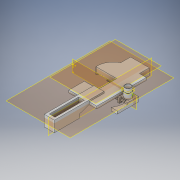
# Autodesk Inventor part: chuteandblocker20200305
Saved by Autodesk Inventor 2018 (Build 220112000, 112)
## iProperties
Created: 2017-08-23
Part Number: chuteandblocker20200305
Material: Generic
Document SubType Name: Modeling
Designer: Kim
Density: 1 g/cm^3
Appearance: Default
Author: Kim
Autodesk Inventor part; units mm, degrees
ref_plane "YZ Plane" through (0, 0, 0) normal (1, 0, 0) x (0, 1, 0)
ref_plane "XZ Plane" through (0, 0, 0) normal (0, 1, 0) x (-1, 0, 0)
ref_plane "XY Plane" through (0, 0, 0) normal (0, 0, 1) x (1, 0, 0)
sketch "Sketch1" plane through (0, 0, 0) normal (0, 1, 0) x (-1, 0, 0)
  line L0 (0, 24.7368) -> (-48.52, 24.7368)
  line L1 (-48.52, 24.7368) -> (-48.52, -25.1832)
  line L2 (-48.52, -25.1832) -> (0, -25.1832)
  line L3 (0, -25.1832) -> (0, 24.7368)
  point P0 (0, 0)
  dimension "d0" = 48.52
  dimension "d1" = 49.92
  constraints: 8 end point, 2 parallel, 1 horizontal, 1 perpendicular
  measures "d0" distance of L2.end L1.end
  measures "d1" distance of L1.end L0.end
extrude "Extrusion1" add sketch "Sketch1" along normal blind 2.5
sketch "Sketch2" plane through (0, 2.5, 0) normal (0, 1, 0) x (1, 0, 0)
  line L0 (0, 25.1832) -> (0, -24.7368) projected
  line L1 (0, -9.2266) -> (34.56, -9.2266)
  line L2 (34.56, -9.2266) -> (34.56, 9.3534)
  line L3 (34.56, 9.3534) -> (0, 9.3534)
  line L4 (0, 9.3534) -> (0, -9.2266)
  point P0 (0, 0)
  dimension "d4" = 34.56
  dimension "d5" = 18.58
  constraints: 8 end point, 2 parallel, 1 horizontal, 1 perpendicular, 1 point on line
  measures "d4" distance of L3.end L2.end
  measures "d5" distance of L2.end L1.end
extrude "Extrusion2" cut sketch "Sketch2" against normal blind 4.25
sketch "Sketch3" plane through (0, 0, 0) normal (0, -1, 0) x (1, 0, 0)
  line L0 (48.52, 24.7368) -> (48.52, -25.1832) projected
  line L1 (48.52, -7.2619) -> (43.52, -7.2619)
  line L2 (43.52, -7.2619) -> (43.52, 1.7381)
  line L3 (43.52, 1.7381) -> (48.52, 1.7381)
  line L4 (48.52, 1.7381) -> (48.52, -7.2619)
  point P0 (0, 0)
  dimension "d8" = 5
  dimension "d9" = 9
  constraints: 8 end point, 2 parallel, 1 horizontal, 1 perpendicular, 1 point on line
  measures "d8" distance of L2.end L3.end
  measures "d9" distance of L1.end L2.end
extrude "Extrusion3" add sketch "Sketch3" along normal blind 6.73
sketch "Sketch4" plane through (48.52, 0, -25.1832) normal (1, 0, 0) x (0, 0, -1)
  line L0 (-17.9213, 0) -> (-17.9213, -6.73) projected
  line L1 (-17.9213, -6.73) -> (-26.9213, -6.73) projected
  line L2 (-17.9213, 0) -> (-26.9213, 0)
  line L3 (-26.9213, 0) -> (-26.9213, -6.73)
  line L4 (-26.9213, -6.73) -> (-17.9213, -6.73)
  line L5 (-17.9213, -6.73) -> (-17.9213, 0)
  line L6 (-17.9213, 0) -> (-17.9213, -6.73) projected
  line L7 (-26.9213, 0) -> (-17.9213, 0)
  line L8 (-17.9213, 0) -> (-17.9213, -4.5)
  line L9 (-17.9213, -4.5) -> (-26.9213, -4.5)
  line L10 (-26.9213, -4.5) -> (-26.9213, 0)
  point P0 (-25.1832, 0)
  dimension "d30" = 4.5
  constraints: 16 end point, 4 parallel, 2 horizontal, 2 perpendicular, 1 point on line
  measures "d30" distance of L7.end L8.end
extrude "Extrusion4" add sketch "Sketch4" along normal blind 10.09
sketch "Sketch5" plane through (48.52, 0, 1.7381) normal (0, 1, 0) x (1, 0, 0)
  circle A0 centre (5, 3.955) radius 2.25
  point P0 (-48.52, 1.7381)
  dimension "d14" = 4.5
  constraints: 1 centre point
  measures "d14" diameter of A0
extrude "Extrusion5" cut sketch "Sketch5" against normal blind 10.09
sketch "Sketch6" plane through (43.52, -6.73, 1.7381) normal (0, 0, 1) x (1, 0, 0)
  line L0 (15.09, 0) -> (15.09, 6.73) projected
  line L1 (12.25, 6.73) -> (12.25, 0) projected
  line L2 (7.75, 6.73) -> (7.75, 0) projected
  line L3 (12.25, 0) -> (7.75, 0)
  line L4 (7.75, 0) -> (7.75, 5.79)
  line L5 (7.75, 5.79) -> (12.25, 5.79)
  line L6 (12.25, 5.79) -> (12.25, 0)
  point P0 (-43.52, 6.73)
  dimension "d19" = 5.79
  constraints: 8 end point, 2 parallel, 1 horizontal, 1 perpendicular, 1 point on line
  measures "d19" distance of L3.end L4.end
extrude "Extrusion6" cut sketch "Sketch6" against normal blind 4.09
sketch "Sketch7" plane through (0, 0, 24.7368) normal (0, 0, 1) x (1, 0, 0)
  line L0 (40.93, 4) -> (30.73, 4)
  line L1 (30.73, 4) -> (30.73, -7)
  line L2 (30.73, -7) -> (40.93, -7)
  line L3 (40.93, -7) -> (40.93, 4)
  point P0 (0, 0)
  dimension "d22" = 10.2
  dimension "d23" = 11
  constraints: 8 end point, 2 parallel, 1 horizontal, 1 perpendicular
  measures "d22" distance of L2.end L1.end
  measures "d23" distance of L1.end L0.end
extrude "Extrusion7" add sketch "Sketch7" along normal blind 35
sketch "Sketch8" plane through (0, 2.5, 0) normal (0, 1, 0) x (1, 0, 0)
  line L0 (33.73, -27.4633) -> (37.93, -27.4633)
  line L1 (37.93, -27.4633) -> (37.93, -56.4633)
  line L2 (37.93, -56.4633) -> (33.73, -56.4633)
  line L3 (33.73, -56.4633) -> (33.73, -27.4633)
  point P0 (0, 0)
  dimension "d26" = 4.2
  dimension "d27" = 29
  constraints: 8 end point, 2 parallel, 1 horizontal, 1 perpendicular
  measures "d26" distance of L1.end L2.end
  measures "d27" distance of L0.end L1.end
extrude "Extrusion8" cut sketch "Sketch8" along normal mid plane 40
sketch "Sketch10" plane through (0, -6.73, 0) normal (0, -1, 0) x (1, 0, 0)
  line L0 (43.52, 1.7381) -> (43.52, -7.2619) projected
  line L1 (58.61, -7.2619) -> (58.61, 1.7381) projected
  line L2 (43.52, 1.7381) -> (58.61, 1.7381)
  line L3 (58.61, 1.7381) -> (58.61, -7.2619)
  line L4 (58.61, -7.2619) -> (43.52, -7.2619)
  line L5 (43.52, -7.2619) -> (43.52, 1.7381)
  point P0 (0, 0)
  constraints: 8 end point, 2 parallel, 1 horizontal, 1 perpendicular
extrude "Extrusion9" cut sketch "Sketch10" against normal blind 2
sketch "Sketch11" plane through (0, 0, 24.7368) normal (0, 0, -1) x (-1, 0, 0)
  line L0 (-30.73, 4) -> (-30.73, -7) projected
  line L1 (-40.93, -7) -> (-40.93, 4) projected
  line L2 (-30.73, -7) -> (-40.93, -7)
  line L3 (-40.93, -7) -> (-40.93, -3.3168)
  line L4 (-40.93, -3.3168) -> (-30.73, -3.3168)
  line L5 (-30.73, -3.3168) -> (-30.73, -7)
  point P0 (0, 0)
  constraints: 8 end point, 2 parallel, 1 horizontal, 1 perpendicular, 1 point on line
extrude "Extrusion10" cut sketch "Sketch11" against normal blind 10
sketch "Sketch13" plane through (0, 2.5, 0) normal (0, 1, 0) x (1, 0, 0)
  arc A0 (6.52, -9.2266) -> (13.0061, -24.7368) centre (31.9994, -7.6829) ccw
  line L0 (0, -9.2266) -> (0, -24.7368) projected
  line L1 (6.52, -9.2266) -> (0, -9.2266)
  line L2 (0, -9.2266) -> (0, -24.7368)
  line L3 (0, -24.7368) -> (13.0061, -24.7368)
  point P0 (0, 0)
  point P1 (48.52, -24.7368)
  constraints: 6 end point, 2 perpendicular, 2 point on circle, 1 centre point, 1 collinear
extrude "Extrusion11" cut sketch "Sketch13" against normal blind 3
sketch "Sketch14" plane through (0, 2.5, 0) normal (0, 1, 0) x (1, 0, 0)
  line L0 (0, 25.1832) -> (0, 9.3534) projected
  line L1 (0, 9.3534) -> (21.0147, 9.3534)
  line L2 (21.0147, 9.3534) -> (21.0147, 25.1832)
  line L3 (21.0147, 25.1832) -> (0, 25.1832)
  line L4 (0, 25.1832) -> (0, 9.3534)
  point P0 (0, 0)
  constraints: 8 end point, 2 parallel, 1 horizontal, 1 perpendicular
extrude "Extrusion12" cut sketch "Sketch14" against normal blind 3
sketch "Sketch15" plane through (48.52, 0, 1.7381) normal (0, 1, 0) x (1, 0, 0)
  circle A0 centre (5, 3.955) radius 2.25 projected
  circle A1 centre (5, 3.955) radius 2.4468
  circle A2 centre (5, 3.955) radius 3.045
  point P0 (-48.52, 1.7381)
  dimension "d42" = 6.09
  constraints: 2 centre point, 2 coincident
  measures "d42" diameter of A2
extrude "Extrusion13" add sketch "Sketch15" along normal blind 2 contours A1 | A2
sketch "Sketch16" plane through (0, 2.5, 0) normal (0, 1, 0) x (1, 0, 0)
  line L0 (6.52, -9.2266) -> (34.56, -9.2266) projected
  arc A0 (6.52, -6.442) -> (20.54, -9.2266) centre (20.7924, 28.7318) ccw
  line L1 (6.52, -6.442) -> (6.52, -9.2266)
  line L2 (6.52, -9.2266) -> (20.54, -9.2266)
  point P0 (0, 0)
  constraints: 4 end point, 2 point on circle, 1 centre point, 1 collinear, 1 midpoint, 1 perpendicular
extrude "Extrusion14" add sketch "Sketch16" against normal blind 2.5
sketch "Sketch17" plane through (0, -4.73, 0) normal (0, -1, 0) x (1, 0, 0)
  arc A0 (51.2741, -2.3519) -> (55.7659, -2.3519) centre (53.52, -2.2169) ccw projected
  line L0 (51.2741, -2.3519) -> (50.4836, 1.7381)
  line L1 (48.52, 1.7381) -> (58.61, 1.7381) projected
  line L2 (50.4836, 1.7381) -> (51.2741, 1.7381)
  line L3 (51.27, -2.3519) -> (51.2741, -2.3519) projected
  line L4 (51.2741, 1.7381) -> (51.2741, -2.3519)
  line L5 (51.2741, -2.3519) -> (50.4836, 1.7381)
  point P0 (0, 0)
  constraints: 8 end point, 1 collinear, 1 horizontal, 1 perpendicular, 1 point on line
extrude "Extrusion15" cut sketch "Sketch17" against normal blind 3.8
sketch "Sketch18" plane through (48.52, 0, 1.7381) normal (0, 1, 0) x (1, 0, 0)
  arc A0 (2.7541, 4.09) -> (2.7541, 3.82) centre (5, 3.955) ccw projected
  line L0 (5, 3.955) -> (7.25, 3.955)
  point P0 (-48.52, 1.7381)
  constraints: 2 end point, 1 horizontal
ref_plane "Work Plane1" through (53.52, 0, -2.2169) normal (0, 0, 1) x (1, 0, 0)
sketch "Sketch19" plane through (53.52, 0, -2.2169) normal (0, 0, 1) x (1, 0, 0)
  line L0 (-2.2459, -4.73) -> (2.2459, -4.73) projected
  line L1 (2.25, 2) -> (2.25, -0.94) projected
  line L2 (2.2459, -4.73) -> (2.25, 2)
  line L3 (2.25, 2) -> (3.045, 1.9995)
  line L4 (3.045, 0) -> (3.045, 2) projected
  line L5 (3.045, 1.9995) -> (2.2459, -4.73)
  line L6 (0, -4.73) -> (0, 1.9995)
  point P0 (-53.52, 0)
  constraints: 8 end point, 1 midpoint, 1 perpendicular, 1 point on line, 1 vertical
sketch "Sketch20" plane through (53.52, 2, -2.2169) normal (0, 1, 0) x (1, 0, 0)
  circle A0 centre (0, 0) radius 3.045
  point P0 (-53.52, -2.2169)
  constraints: 1 centre point
sketch "Sketch21" plane through (0, -4.73, 0) normal (0, -1, 0) x (1, 0, 0)
  circle A0 centre (53.5206, 0.0446) radius 2.2507
  point P0 (0, 0)
  constraints: 1 centre point
loft "Loft1" cut profiles "Sketch21" section 1 edges at (50.475, 2, -2.2169)
sketch "Sketch22" plane through (43.52, 0, 1.7381) normal (0, 0, 1) x (1, 0, 0)
  line L0 (12.25, -4.73) -> (12.25, -4.73) projected
  line L1 (15.09, -4.73) -> (15.09, 0) projected
  line L2 (12.2474, -4.73) -> (15.09, -4.73)
  line L3 (15.09, -4.73) -> (15.09, -1.73)
  line L4 (15.09, -1.73) -> (12.2474, -1.73)
  line L5 (12.2474, -1.73) -> (12.2474, -4.73)
  point P0 (-43.52, 0)
  point P1 (7.7539, -4.73)
  dimension "d54" = 3
  constraints: 8 end point, 2 parallel, 1 horizontal, 1 perpendicular, 1 point on line, 1 other
  measures "d54" distance of L3.end L2.end
extrude "Extrusion16" add sketch "Sketch22" along normal blind 10
sketch "Sketch23" plane through (43.52, 0, 1.7381) normal (0, 0, 1) x (1, 0, 0)
  line L0 (7.75, -4.73) -> (6.9636, -4.73) projected
  line L1 (6.9636, -4.73) -> (4.9636, -4.73)
  line L2 (4.9636, -4.73) -> (4.9636, -1.73)
  line L3 (4.9636, -1.73) -> (6.9636, -1.73)
  line L4 (6.9636, -1.73) -> (6.9636, -4.73)
  point P0 (-43.52, 0)
  dimension "d57" = 2
  dimension "d58" = 3
  constraints: 8 end point, 2 parallel, 1 horizontal, 1 perpendicular
  measures "d57" distance of L2.end L3.end
  measures "d58" distance of L1.end L2.end
extrude "Extrusion17" add sketch "Sketch23" along normal blind 2
sketch "Sketch24" plane through (55.77, -1.73, 1.7381) normal (0, 1, 0) x (1, 0, 0)
  line L0 (-4.4959, 0) -> (0, 0) projected
  line L1 (2.84, 9) -> (2.84, -10) projected
  line L2 (0, 0) -> (2.84, 0)
  line L3 (2.84, 0) -> (2.84, -1)
  line L4 (2.84, -1) -> (0, -1)
  line L5 (0, -1) -> (0, 0)
  line L6 (0, -1) -> (2.84, -1)
  line L7 (2.84, -1) -> (2.84, -2)
  line L8 (2.84, -2) -> (0, -2)
  line L9 (0, -2) -> (0, -1)
  point P0 (-55.77, 1.7381)
  dimension "d61" = 1
  dimension "d62" = 1
  constraints: 16 end point, 4 parallel, 2 horizontal, 2 perpendicular, 2 point on line
  measures "d61" distance of L2.end L3.end
  measures "d62" distance of L6.end L7.end
extrude "Extrusion18" add sketch "Sketch24" along normal blind 1.75 contours L1 L8 L9 L4
sketch "Sketch25" plane through (48.4836, -1.73, 1.7381) normal (0, 1, 0) x (1, 0, 0)
  line L0 (0, 0) -> (2, 0) projected
  line L1 (0, 0) -> (0, -2) projected
  line L2 (2, 0) -> (0, 0)
  line L3 (0, 0) -> (0, -1)
  line L4 (0, -1) -> (2, -1)
  line L5 (2, -1) -> (2, 0)
  line L6 (2, -2) -> (0, -2) projected
  line L7 (2, -1) -> (0, -1)
  line L8 (0, -1) -> (0, -2)
  line L9 (0, -2) -> (2, -2)
  line L10 (2, -2) -> (2, -1)
  point P0 (-48.4836, 1.7381)
  dimension "d65" = 1
  constraints: 16 end point, 4 parallel, 2 horizontal, 2 perpendicular, 1 midpoint
  measures "d65" distance of L3.end L2.end
extrude "Extrusion19" add sketch "Sketch25" along normal blind 1.75 contours L4 L10 L6 L1
sketch "Sketch26" plane through (58.61, -1.73, 2.7381) normal (0, 0, -1) x (-1, 0, 0)
  line L0 (0, 0) -> (0, 1.75) projected
  line L1 (2.84, 0) -> (0, 0)
  line L2 (0, 0) -> (0, 0.5)
  line L3 (0, 0.5) -> (2.84, 0.5)
  line L4 (2.84, 0.5) -> (2.84, 0)
  line L5 (2.84, 0.5) -> (0, 0.5)
  line L6 (0, 0.5) -> (0, 1.75)
  line L7 (0, 1.75) -> (2.84, 1.75)
  line L8 (2.84, 1.75) -> (2.84, 0.5)
  point P0 (58.61, 1.73)
  dimension "d68" = 0.5
  constraints: 16 end point, 4 parallel, 2 horizontal, 2 perpendicular, 1 point on line
  measures "d68" distance of L1.end L2.end
extrude "Extrusion20" add sketch "Sketch26" along normal blind 1.2 contours L0 L7 L8 L3
sketch "Sketch27" plane through (50.4836, -1.73, 2.7381) normal (0, 0, -1) x (-1, 0, 0)
  line L0 (2, 0) -> (0, 0) projected
  line L1 (0, 0) -> (0, 1.75) projected
  line L2 (2, 0) -> (0, 0)
  line L3 (0, 0) -> (0, 0.5)
  line L4 (0, 0.5) -> (2, 0.5)
  line L5 (2, 0.5) -> (2, 0)
  line L6 (0, 1.75) -> (1.9636, 1.75) projected
  line L7 (2, 0.5) -> (0, 0.5)
  line L8 (0, 0.5) -> (0, 1.75)
  line L9 (0, 1.75) -> (2, 1.75)
  line L10 (2, 1.75) -> (2, 0.5)
  point P0 (50.4836, 1.73)
  dimension "d71" = 0.5
  constraints: 16 end point, 4 parallel, 2 horizontal, 2 perpendicular, 1 point on line
  measures "d71" distance of L2.end L3.end
extrude "Extrusion21" add sketch "Sketch27" along normal blind 1.2 contours L4 L1 L6 L9 L10
sketch "Sketch28" plane through (21.0147, 2.5, -25.1832) normal (-1, 0, 0) x (0, 0, 1)
  line L0 (0, 0) -> (15.8297, 0) projected
  line L1 (15.8297, -2.5) -> (0, -2.5) projected
  line L2 (0, 0) -> (15.8297, 0)
  line L3 (15.8297, 0) -> (15.8297, -2.5)
  line L4 (15.8297, -2.5) -> (0, -2.5)
  line L5 (0, -2.5) -> (0, 0)
  point P0 (25.1832, -2.5)
  constraints: 8 end point, 2 parallel, 1 horizontal, 1 perpendicular
extrude "Extrusion22" add sketch "Sketch28" along normal blind 9.03
sketch "Sketch29" plane through (0, 2.5, 0) normal (0, 1, 0) x (1, 0, 0)
  line L0 (48.52, 25.1832) -> (11.9847, 25.1832) projected
  line L1 (11.9847, 25.1832) -> (21.0147, 25.1832)
  line L2 (34.56, 9.3534) -> (11.9847, 9.3534) projected
  line L3 (21.0147, 25.1832) -> (11.9847, 9.3534)
  line L4 (11.9847, 9.3534) -> (11.9847, 25.1832)
  point P0 (0, 0)
  dimension "d76" = 9.03
  constraints: 6 end point, 1 perpendicular, 1 point on line
  measures "d76" distance of L0.end L1.end
extrude "Extrusion23" cut sketch "Sketch29" against normal blind 4
sketch "Sketch30" plane through (0, 0, 0) normal (0, -1, 0) x (1, 0, 0)
  line L0 (21.0147, -25.1832) -> (11.9847, -9.3534) projected
  line L1 (34.56, -9.3534) -> (11.9847, -9.3534) projected
  line L2 (11.9847, -9.3534) -> (34.56, -9.3534)
  line L3 (34.56, -9.3534) -> (34.56, -25.1832)
  line L4 (48.52, -25.1832) -> (21.0147, -25.1832) projected
  line L5 (34.56, -25.1832) -> (21.0147, -25.1832)
  line L6 (21.0147, -25.1832) -> (11.9847, -9.3534)
  point P0 (0, 0)
  constraints: 8 end point, 2 collinear, 1 perpendicular, 1 point on line
extrude "Extrusion24" add sketch "Sketch30" along normal blind 2.5
sketch "Sketch31" plane through (0, 0, 0) normal (0, -1, 0) x (1, 0, 0)
  line L0 (34.56, -9.3534) -> (34.56, -25.1832) projected
  line L1 (48.52, -25.1832) -> (21.0147, -25.1832) projected
  line L2 (34.56, -9.3534) -> (41.56, -9.3534)
  line L3 (41.56, -9.3534) -> (41.56, -25.1832)
  line L4 (41.56, -25.1832) -> (34.56, -25.1832)
  line L5 (34.56, -25.1832) -> (34.56, -9.3534)
  point P0 (0, 0)
  dimension "d81" = 7
  constraints: 8 end point, 2 parallel, 1 horizontal, 1 perpendicular, 1 point on line
  measures "d81" distance of L3.end L4.end
extrude "Extrusion25" add sketch "Sketch31" along normal blind 2.5
sketch "Sketch32" plane through (0, -2.5, 0) normal (0, -1, 0) x (1, 0, 0)
  line L0 (41.56, -9.3534) -> (11.9847, -9.3534) projected
  line L1 (21.0147, -25.1832) -> (41.56, -25.1832) projected
  line L2 (41.56, -9.3534) -> (37.56, -9.3534)
  line L3 (37.56, -9.3534) -> (37.56, -25.1832)
  line L4 (37.56, -25.1832) -> (41.56, -25.1832)
  line L5 (41.56, -25.1832) -> (41.56, -9.3534)
  point P0 (0, 0)
  dimension "d84" = 4
  constraints: 8 end point, 2 parallel, 1 horizontal, 1 perpendicular, 1 point on line
  measures "d84" distance of L4.end L3.end
extrude "Extrusion26" add sketch "Sketch32" along normal blind 2
sketch "Sketch33" plane through (37.56, -2.5, -25.1832) normal (-1, 0, 0) x (0, 0, 1)
  line L0 (15.8297, -2) -> (0, -2) projected
  line L1 (15.8297, 2.5) -> (15.8297, -2) projected
  line L2 (0, -2) -> (15.8297, -2)
  line L3 (15.8297, -2) -> (15.8297, -1.25)
  line L4 (15.8297, -1.25) -> (0, -1.25)
  line L5 (0, -1.25) -> (0, -2)
  point P0 (25.1832, 2.5)
  dimension "d87" = 0.75
  constraints: 8 end point, 2 parallel, 1 horizontal, 1 perpendicular, 1 point on line
  measures "d87" distance of L3.end L2.end
extrude "Extrusion27" add sketch "Sketch33" along normal blind 13
sketch "Sketch34" plane through (55.77, -1.73, 1.7381) normal (0, 1, 0) x (1, 0, 0)
  line L0 (-0.0026, 0) -> (-0.0026, -10) projected
  line L1 (0, -1) -> (2.84, -1) projected
  line L2 (-0.0026, 0) -> (2.84, 0)
  line L3 (2.84, 0) -> (2.84, -1)
  line L4 (2.84, -1) -> (-0.0026, -1)
  line L5 (-0.0026, -1) -> (-0.0026, 0)
  point P0 (-55.77, 1.7381)
  constraints: 8 end point, 2 parallel, 1 horizontal, 1 perpendicular
extrude "Extrusion28" cut sketch "Sketch34" against normal blind 1
sketch "Sketch35" plane through (48.4836, -1.73, 1.7381) normal (0, 1, 0) x (1, 0, 0)
  line L0 (2, -1) -> (2, 0) projected
  line L1 (0, -1) -> (0, 0) projected
  line L2 (2, -1) -> (0, -1)
  line L3 (0, -1) -> (0, 0)
  line L4 (0, 0) -> (2, 0)
  line L5 (2, 0) -> (2, -1)
  point P0 (-48.4836, 1.7381)
  constraints: 8 end point, 2 parallel, 1 horizontal, 1 perpendicular
extrude "Extrusion29" cut sketch "Sketch35" against normal blind 1
sketch "Sketch36" plane through (0, 2.5, 0) normal (0, 1, 0) x (1, 0, 0)
  line L0 (48.52, 25.1832) -> (21.0147, 25.1832) projected
  line L1 (11.9847, 9.3534) -> (34.56, 9.3534) projected
  arc A0 (21.0147, 25.1832) -> (11.9847, 9.3534) centre (27.923, 10.7519) ccw
  line L2 (21.0147, 25.1832) -> (11.9847, 9.3534)
  point P0 (0, 0)
  constraints: 2 end point, 2 point on circle, 1 centre point
extrude "Extrusion30" add sketch "Sketch36" against normal blind 7
sketch "Sketch37" plane through (0, 0, 24.7368) normal (0, 0, -1) x (-1, 0, 0)
  line L0 (-40.93, 2.5) -> (-40.93, 4) projected
  line L1 (-30.73, 4) -> (-30.73, -7) projected
  line L2 (-40.93, 4) -> (-30.73, 4)
  line L3 (-30.73, 4) -> (-30.73, 2.4982)
  line L4 (-30.73, 2.4982) -> (-40.93, 2.4982)
  line L5 (-40.93, 2.4982) -> (-40.93, 4)
  point P0 (0, 0)
  constraints: 8 end point, 2 parallel, 1 horizontal, 1 perpendicular, 1 point on line
extrude "Extrusion31" add sketch "Sketch37" along normal blind 15
sketch "Sketch38" plane through (48.52, 0, -25.1832) normal (0, 0, -1) x (-1, 0, 0)
  line L0 (27.5053, 2.5) -> (27.5053, -2.5) projected
  line L1 (6.96, 0) -> (6.96, -4.5) projected
  line L2 (27.5053, 2.5) -> (6.96, 2.5)
  line L3 (6.96, 2.5) -> (6.96, -2.4833)
  line L4 (6.96, -2.4833) -> (27.5053, -2.4833)
  line L5 (27.5053, -2.4833) -> (27.5053, 2.5)
  point P0 (48.52, 0)
  constraints: 8 end point, 2 parallel, 1 horizontal, 1 perpendicular, 1 point on line
extrude "Extrusion32" add sketch "Sketch38" along normal blind 10
sketch "Sketch39" plane through (21.0147, -2.4833, -25.1832) normal (0, -1, 0) x (1, 0, 0)
  line L0 (0, -10) -> (20.5453, -10) projected
  line L1 (20.5453, 0) -> (20.5453, -10) projected
  line L2 (0, -10) -> (20.5453, -10)
  line L3 (20.5453, -10) -> (20.5453, -0.2764)
  line L4 (20.5453, -0.2764) -> (0, -0.2764)
  line L5 (0, -0.2764) -> (0, -10)
  point P0 (-21.0147, 25.1832)
  constraints: 8 end point, 2 parallel, 1 horizontal, 1 perpendicular, 1 point on line
extrude "Extrusion33" add sketch "Sketch39" along normal blind 2
ref_plane "Work Plane2" through (0, 7.175, 0) normal (0, 1, 0) x (1, 0, 0)
sketch "Sketch40" plane through (0, 7.175, 0) normal (0, 1, 0) x (1, 0, 0)
  circle A0 centre (53.5373, 1.7566) radius 3.1004
  circle A1 centre (53.5373, 1.7566) radius 2.7105
  point P0 (0, 0)
  constraints: 2 centre point, 1 coincident
sketch "Sketch41" plane through (0, -4.73, 0) normal (0, -1, 0) x (1, 0, 0)
  arc A0 (51.2284, 0.045) -> (55.7687, 0.045) centre (53.4986, 0.045) ccw
  arc A1 (50.475, 0.045) -> (56.565, 0.045) centre (53.52, 0.045) ccw
  line L0 (56.565, 0.045) -> (55.7687, 0.045)
  line L1 (51.2284, 0.045) -> (50.475, 0.045)
  point P0 (0, 0)
  constraints: 5 point on circle, 4 end point, 2 centre point, 1 coincident, 1 horizontal
extrude "Extrusion34" add sketch "Sketch40" against normal blind 8
ref_plane "Work Plane3" through (39.43, 0, 24.7368) normal (1, 0, 0) x (0, 0, -1)
sketch "Sketch42" plane through (39.43, 0, 24.7368) normal (1, 0, 0) x (0, 0, -1)
  line L0 (0, 0) -> (0, -3.3168) projected
  line L1 (-10, -3.3168) -> (0, -3.3168)
  line L2 (0, -3.3168) -> (0, 0)
  line L3 (-2.7264, -3.3168) -> (-10, -3.3168) projected
  line L4 (0, 0) -> (-10, -3.3168)
  line L5 (-10, -3.3168) -> (0, 0)
  point P0 (24.7368, 0)
  constraints: 8 end point, 2 collinear, 1 horizontal
extrude "Extrusion35" cut sketch "Sketch42" along normal mid plane 40
ref_plane "Work Plane4" through (0, 1.25, 0) normal (0, 1, 0) x (1, 0, 0)
sketch "Sketch43" plane through (0, 1.25, 0) normal (0, 1, 0) x (1, 0, 0)
  line L0 (20.54, -9.2266) -> (20.54, -24.7368)
  line L1 (20.54, -24.7368) -> (4.0668, -24.7368)
  line L2 (4.0668, -24.7368) -> (4.0668, -5.638)
  line L3 (4.0668, -5.638) -> (20.54, -5.638)
  line L4 (20.54, -5.638) -> (20.54, -9.2266)
  line L5 (20.54, -9.2266) -> (20.54, -24.7368)
  point P0 (0, 0)
  constraints: 12 end point, 3 perpendicular, 1 collinear, 1 horizontal, 1 point on line, 1 vertical
extrude "Extrusion36" cut sketch "Sketch43" along normal mid plane 20
ref_plane "Work Plane5" through (53.5373, 7.175, -1.7566) normal (0, 1, 0) x (1, 0, 0)
sketch "Sketch44" plane through (53.5373, 7.175, -1.7566) normal (0, 1, 0) x (1, 0, 0)
  circle A0 centre (0, 0) radius 2.7105 projected
  circle A1 centre (0, 0) radius 2.7105
  circle A2 centre (0, 0) radius 3.1004
  point P0 (-53.5373, -1.7566)
  constraints: 2 centre point, 2 coincident
extrude "Extrusion37" add sketch "Sketch44" along normal blind 2
sketch "Sketch45" plane through (0, 2.5, 0) normal (0, 1, 0) x (1, 0, 0)
  arc A0 (22.7812, 25.1466) -> (13.7632, 9.3583) centre (29.7045, 10.7225) ccw
  line L0 (22.7812, 25.1466) -> (22.7812, 35.1832)
  line L1 (20.5792, 35.5788) -> (19.838, 25.3776)
  line L2 (21.0147, 25.4596) -> (21.0147, 35.1832) projected
  line L3 (19.838, 25.3776) -> (10.2515, 25.3776)
  line L4 (10.2515, 25.3776) -> (10.2515, 9.0553)
  line L5 (10.2515, 9.0553) -> (13.7632, 9.3583)
  line L6 (22.7812, 35.1832) -> (20.5792, 35.5788)
  point P0 (0, 0)
  constraints: 10 end point, 2 point on circle, 2 vertical, 1 centre point, 1 horizontal, 1 perpendicular, 3 other
extrude "Extrusion40" cut sketch "Sketch45" against normal blind 10
sketch "Sketch46" plane through (0, -4.5, 0) normal (0, -1, 0) x (1, 0, 0)
  line L0 (22.7812, -25.1832) -> (41.56, -25.1832) projected
  line L1 (13.7064, -9.3534) -> (34.56, -9.3534) projected
  line L2 (22.7812, -25.1832) -> (13.7064, -9.3534)
  arc A0 (13.7064, -9.3534) -> (22.7812, -25.1832) centre (29.914, -10.578) ccw
  point P0 (0, 0)
  constraints: 2 end point, 2 point on circle, 1 centre point
extrude "Extrusion41" add sketch "Sketch46" against normal blind 7
sketch "Sketch47" plane through (55.7674, -1.73, 11.7381) normal (0, 1, 0) x (1, 0, 0)
  arc A0 (-3.1282, -2.5889) -> (0.0026, 10) centre (-21.5677, 8.6808) ccw
  line L0 (-3.1282, -2.5889) -> (2.8426, -2.5889)
  line L1 (2.8426, 8) -> (0.0026, 8)
  line L2 (2.8426, -2.5889) -> (2.8426, 10.1735)
  line L3 (0.0026, 10) -> (2.8426, 10) projected
  line L4 (2.8426, 19) -> (2.8426, 10.2) projected
  line L5 (2.8426, 10.1735) -> (2.8426, 10.2)
  line L6 (0.0026, 11.6144) -> (0.0026, 10) projected
  line L7 (2.8426, 10.2) -> (0.0026, 10)
  point P0 (-55.7674, 11.7381)
  constraints: 10 end point, 2 point on circle, 1 centre point, 1 collinear, 1 horizontal, 1 perpendicular
extrude "Extrusion42" add sketch "Sketch47" against normal blind 3
sketch "Sketch48" plane through (48.4836, -4.73, 3.7381) normal (-1, 0, 0) x (0, 0, 1)
  line L0 (-1, 3.5) -> (-2, 3.5) projected
  line L1 (-2, 2) -> (-2, 0) projected
  line L2 (-1, 3.5) -> (-2, 3.5)
  line L3 (-2, 3.5) -> (-2, 2)
  line L4 (-2, 2) -> (-1, 2)
  line L5 (-1, 2) -> (-1, 3.5)
  point P0 (-3.7381, 4.73)
  constraints: 8 end point, 2 parallel, 1 horizontal, 1 perpendicular
extrude "Extrusion43" cut sketch "Sketch48" against normal blind 15
sketch "Sketch49" plane through (58.61, 0, -25.1832) normal (1, 0, 0) x (0, 0, -1)
  line L0 (-27.9213, -1.23) -> (-27.9213, -2.73) projected
  line L1 (-26.9213, -2.73) -> (-26.9213, -1.23) projected
  line L2 (-27.9213, -2.73) -> (-26.9213, -2.73)
  line L3 (-26.9213, -2.73) -> (-26.9213, -1.23)
  line L4 (-26.9213, -1.23) -> (-27.9213, -1.23)
  line L5 (-27.9213, -1.23) -> (-27.9213, -2.73)
  point P0 (-25.1832, 0)
  constraints: 8 end point, 2 parallel, 1 horizontal, 1 perpendicular
extrude "Extrusion44" add sketch "Sketch49" against normal blind 10.1
ref_plane "Work Plane6" through (53.5373, 5.175, -1.7566) normal (0, 1, 0) x (1, 0, 0)
sketch "Sketch50" plane through (53.5373, 5.175, -1.7566) normal (0, 1, 0) x (1, 0, 0)
  circle A0 centre (0, 0) radius 3.093
  circle A1 centre (0, 0) radius 3.4145
  point P0 (-53.5373, -1.7566)
  constraints: 2 centre point, 1 coincident
extrude "Extrusion45" add sketch "Sketch50" against normal blind 5.5
sketch "Sketch51" plane through (30.73, 4, 59.7368) normal (0, 1, 0) x (1, 0, 0)
  line L0 (2.3064, 32.2736) -> (7.9046, 32.2736)
  line L1 (7.9046, 32.2736) -> (7.9046, 2.8217)
  line L2 (7.9046, 2.8217) -> (2.3064, 2.8217)
  line L3 (2.3064, 2.8217) -> (2.3064, 32.2736)
  point P0 (-30.73, 59.7368)
  constraints: 8 end point, 2 parallel, 1 horizontal, 1 perpendicular
extrude "Extrusion46" cut sketch "Sketch51" against normal blind 15
body "Solid1"
